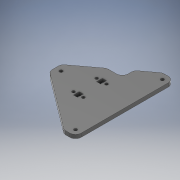
# Autodesk Inventor part: Y_Axis_Carriage_Plate_LM3039
Saved by Autodesk Inventor 2020.3 (Build 243373000, 373)
## iProperties
Created: 2020-05-30
Part Number: Y_Axis_Carriage_Plate_LM3039
Material: Acetal Resin, Black
Document SubType Name: Modeling
Designer: rah75
Density: 1.425 g/cm^3
Appearance: Smooth - Black
Author: rah75
Autodesk Inventor part; units mm, degrees
ref_plane "YZ Plane" through (0, 0, 0) normal (1, 0, 0) x (0, 1, 0)
ref_plane "XZ Plane" through (0, 0, 0) normal (0, 1, 0) x (-1, 0, 0)
ref_plane "XY Plane" through (0, 0, 0) normal (0, 0, 1) x (1, 0, 0)
sketch "Sketch1" plane through (0, 0, 0) normal (0, 1, 0) x (-1, 0, 0)
  line L0 (10, -85) -> (110, -10)
  line L1 (110, -10) -> (110, 10)
  line L2 (110, 10) -> (10, 85)
  line L3 (10, 85) -> (-10, 85)
  line L4 (-10, 85) -> (-10, -85)
  line L5 (-10, -85) -> (10, -85)
  point P0 (0, 0)
  point P1 (100, 0)
  point P2 (0, -75)
  point P3 (0, 75)
  point P4 (-10, 0)
  point P5 (110, 0)
  dimension "d0" = 170
  dimension "d1" = 100
  dimension "d2" = 150
  dimension "d3" = 75
  dimension "d4" = 10
  dimension "d5" = 10
  dimension "d6" = 36.87
  dimension "d7" = 20
  dimension "d8" = 20
  constraints: 12 end point, 3 horizontal alignment, 3 perpendicular, 2 midpoint, 2 vertical alignment, 1 parallel, 1 vertical
  measures "d0" distance of L3.end L4.end
  measures "d1" horizontal distance of point (0, -75) point (100, 0)
  measures "d2" distance of point (0, 75) point (0, -75)
  measures "d3" distance of point (0, 0) point (0, -75)
  measures "d4" distance from line of L4 point (0, -75)
  measures "d5" distance from line of L1 point (100, 0)
  measures "d6" angle of L0 L5
  measures "d7" distance of L4.end L0.start
  measures "d8" distance of L0.end L1.end
extrude "Extrusion1" add sketch "Sketch1" along normal mid plane 6.35
fillet "Fillet1" radius 10 6 edges at (-10, 0, 85) (10, 0, 85) (10, 0, -85) (-10, 0, -85) (-110, 0, -10) (-110, 0, 10)
sketch "Sketch2" plane through (0, 3.175, 0) normal (0, 1, 0) x (1, 0, 0)
  arc A0 (0, -85) -> (10, -75) centre (0, -75) ccw projected
  arc A1 (10, 75) -> (0, 85) centre (0, 75) ccw projected
  line L0 (-110, 5) -> (-110, -5) projected
  point P0 (0, 0)
  point P1 (-100, 0)
  dimension "d12" = 10
  constraints: 1 horizontal alignment
  measures "d12" distance from line of point (-100, 0) L0
hole "Hole1" at (-100, 3.175, 0) at (0, 3.175, -75) at (0, 3.175, 75) direction (0, -1, 0) diameter 5.5 depth 7.6 tip angle 118 start extended yes
sketch "Sketch3" plane through (0, 3.175, 0) normal (0, 1, 0) x (1, 0, 0)
  circle A0 centre (-100, 0) radius 2.75 projected
  line L0 (-65, 43.75) -> (-38, 43.75)
  line L1 (-38, 43.75) -> (-38, 64)
  line L2 (-38, 64) -> (-65, 43.75)
  line L3 (-12.6667, 83) -> (-106, 13) projected
  point P0 (0, 0)
  dimension "d20" = 35
  dimension "d21" = 27
  constraints: 6 end point, 1 collinear, 1 horizontal, 1 vertical
  measures "d20" horizontal distance of A0.centre L0.start
  measures "d21" distance of L0.start L0.end
extrude "Extrusion2" cut sketch "Sketch3" against normal blind 10 contours L2 L1 L0
fillet "Fillet2" radius 10 3 edges at (-65, 0, -43.75) (-38, 0, -43.75) (-38, 0, -64)
sketch "Sketch4" plane through (0, -3.175, 0) normal (0, -1, 0) x (1, 0, 0)
  line L0 (-58.5, -20) -> (-41.5, -20)
  line L1 (0, 0) -> (-6.0642, 0)
  point P0 (-50, -20)
  point P1 (-58.5, 20)
  point P2 (-41.5, 20)
  point P3 (-50, 20)
  dimension "d25" = 50
  dimension "d26" = 17
  dimension "d27" = 20
  constraints: 4 end point, 3 symmetric about line, 2 coincident, 2 horizontal, 1 midpoint
  measures "d25" horizontal distance of point (-50, -20) L1.start
  measures "d26" distance of L0.start L0.end
  measures "d27" distance from line of L1.start L0
hole "Hole2" at (-58.5, -3.175, -20) at (-41.5, -3.175, -20) at (-41.5, -3.175, 20) at (-58.5, -3.175, 20) at (-50, -3.175, -20) at (-50, -3.175, 20) direction (0, 1, 0) diameter 5 end through all
sketch "Sketch5" plane through (0, 3.175, 0) normal (0, 1, 0) x (1, 0, 0)
  circle A0 centre (-50, 20) radius 2.5 projected
  circle A1 centre (-41.5, -20) radius 2.5 projected
  circle A2 centre (-58.5, 20) radius 2.5 projected
  circle A3 centre (-41.5, 20) radius 2.5 projected
  circle A4 centre (-58.5, -20) radius 2.5 projected
  circle A5 centre (-50, -20) radius 2.5 projected
  arc A6 (-34, 67) -> (-38, 59) centre (-28, 59) ccw projected
  line L0 (-38, 59) -> (-38, 53.75) projected
  arc A7 (-48, 43.75) -> (-38, 53.75) centre (-48, 53.75) ccw projected
  line L1 (-48, 43.75) -> (-61.6667, 43.75) projected
  arc A8 (-61.6667, 43.75) -> (-67.6667, 41.75) centre (-61.6667, 33.75) ccw projected
  line L2 (-67.6667, 41.75) -> (-106, 13) projected
  arc A9 (-106, 13) -> (-110, 5) centre (-100, 5) ccw projected
  line L3 (-110, 5) -> (-110, -5) projected
  arc A10 (-110, -5) -> (-106, -13) centre (-100, -5) ccw projected
  line L4 (-106, -13) -> (-12.6667, -83) projected
  arc A11 (-12.6667, -83) -> (-6.6667, -85) centre (-6.6667, -75) ccw projected
  line L5 (-6.6667, -85) -> (0, -85) projected
  arc A12 (0, -85) -> (10, -75) centre (0, -75) ccw projected
  line L6 (10, -75) -> (10, 75) projected
  arc A13 (10, 75) -> (0, 85) centre (0, 75) ccw projected
  line L7 (0, 85) -> (-6.6667, 85) projected
  arc A14 (-6.6667, 85) -> (-12.6667, 83) centre (-6.6667, 75) ccw projected
  line L8 (-12.6667, 83) -> (-34, 67) projected
  circle A15 centre (0, 75) radius 2.75 projected
  circle A16 centre (-100, 0) radius 2.75 projected
  circle A17 centre (0, -75) radius 2.75 projected
  line L9 (-53.5, 25) -> (-46.5, 25)
  line L10 (-46.5, 25) -> (-46.5, 15)
  line L11 (-46.5, 15) -> (-53.5, 15)
  line L12 (-53.5, 15) -> (-53.5, 25)
  line L13 (-53.5, 25) -> (-46.5, 15) construction
  line L14 (-46.5, 25) -> (-53.5, 15) construction
  line L15 (-53.5, -15) -> (-46.5, -15)
  line L16 (-46.5, -15) -> (-46.5, -25)
  line L17 (-46.5, -25) -> (-53.5, -25)
  line L18 (-53.5, -25) -> (-53.5, -15)
  line L19 (-53.5, -15) -> (-46.5, -25) construction
  line L20 (-46.5, -15) -> (-53.5, -25) construction
  point P0 (0, 0)
  dimension "d35" = 7
  dimension "d36" = 10
  dimension "d37" = 7
  dimension "d38" = 10
  constraints: 24 end point, 4 midpoint, 4 parallel, 2 horizontal, 2 perpendicular
  measures "d35" distance of L10.end L11.end
  measures "d36" distance of L9.end L10.end
  measures "d37" distance of L16.end L17.end
  measures "d38" distance of L15.end L16.end
extrude "Extrusion3" cut sketch "Sketch5" against normal blind 10 contours A0 | A5 | L9 L10 L11 L12 | L15 L16 L17 L18
body "Solid1"
